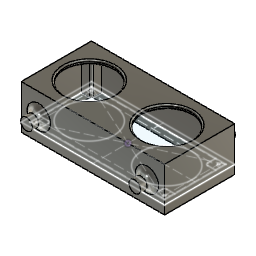
Soporte_EspejoRetrovisor v10 (Autodesk Fusion 360 archive; units mm, degrees)
design "HC-SR04"
Autodesk Fusion 360 part; units mm, degrees
sketch "Boceto1" plane through (0, 0, 0) normal (0, 0, 1) x (1, 0, 0)
  line L0 (22.75, 10.25) -> (-22.75, 10.25)
  line L1 (-22.75, 10.25) -> (-22.75, -10.25)
  line L2 (-22.75, -10.25) -> (22.75, -10.25)
  line L3 (22.75, -10.25) -> (22.75, 10.25)
  line L4 (22.75, 10.25) -> (-22.75, -10.25) construction
  line L5 (-22.75, 10.25) -> (22.75, -10.25) construction
  line L6 (-22.75, -8.5) -> (22.75, -8.5) construction
  line L7 (-21.75, 10.25) -> (-21.75, -10.25) construction
  line L8 (21.75, 10.25) -> (21.75, -10.25) construction
  line L9 (-22.75, 8.5) -> (22.75, 8.5) construction
  circle A0 centre (13.25, 0) radius 8.5
  circle A1 centre (-21.75, 9.25) radius 1 construction
  circle A2 centre (-21.75, 9.25) radius 0.5
  line L10 (12.75, 6.5) -> (22.75, 6.5) construction
  line L11 (0, 10.25) -> (0, -10.25) construction
  circle A3 centre (-13.25, 0) radius 8.5
  line L12 (-22.75, 0) -> (22.75, 0) construction
  line L13 (-22.75, 7.75) -> (22.75, 7.75) construction
  line L14 (-5.0036, 6) -> (5.0036, 6)
  arc A4 (5.0036, 6) -> (5.0036, 9.5) centre (5.0036, 7.75) ccw
  line L15 (5.0036, 9.5) -> (-5.0036, 9.5)
  arc A5 (-5.0036, 9.5) -> (-5.0036, 6) centre (-5.0036, 7.75) ccw
  line L16 (-5.0036, 7.75) -> (5.0036, 7.75) construction
  circle A6 centre (21.75, 9.25) radius 0.5
  circle A7 centre (21.75, 9.25) radius 1 construction
  circle A8 centre (-21.75, -9.25) radius 0.5
  circle A9 centre (-21.75, -9.25) radius 1 construction
  circle A10 centre (21.75, -9.25) radius 1 construction
  circle A11 centre (21.75, -9.25) radius 0.5
  line L17 (-5.0036, -6) -> (5.0036, -6)
  arc A12 (-5.0036, -6) -> (-5.0036, -9.5) centre (-5.0036, -7.75) ccw
  line L18 (5.0036, -9.5) -> (-5.0036, -9.5)
  arc A13 (5.0036, -9.5) -> (5.0036, -6) centre (5.0036, -7.75) ccw
  dimension "d1" = 45.5
  dimension "d2" = 20.5
  dimension "d4" = 1.75
  dimension "d6" = 1
  dimension "d7" = 1
  dimension "d8" = 1.75
  dimension "d9" = 8.5
  dimension "d23" = 1
  dimension "d24" = -0.5
  dimension "d135" = 2.5
  dimension "d136" = 3.5
  constraint horizontal L0
  constraint perpendicular L0 L1
  constraint parallel L0 L2
  constraint parallel L1 L3
  constraint coincident L4 origin
  constraint coincident L5 origin
  constraint coincident L1 L6.start
  constraint coincident L3 L6.end
  constraint perpendicular L3 L6
  constraint coincident L0 L7.start
  constraint coincident L2 L7.end
  constraint perpendicular L2 L7
  constraint coincident L0 L8.start
  constraint coincident L2 L8.end
  constraint perpendicular L2 L8
  constraint coincident L1 L9.start
  constraint coincident L3 L9.end
  constraint perpendicular L3 L9
  constraint tangent L8 A0
  constraint tangent L6 A0
  constraint tangent L0 A1
  constraint tangent L1 A1
  constraint coincident L3 L10.end
  constraint perpendicular L3 L10
  constraint midpoint L0 L11.start
  constraint midpoint L2 L11.end
  constraint symmetric A0 L11 A3
  constraint midpoint L1 L12.start
  constraint midpoint L3 L12.end
  constraint coincident L1 L13.start
  constraint coincident L3 L13.end
  constraint perpendicular L3 L13
  constraint tangent L14 A4
  constraint tangent A4 L15
  constraint parallel L14 L15
  constraint tangent L15 A5
  constraint tangent L14 A5
  constraint perpendicular L11 L16
  constraint coincident L13 A5.centre
  constraint midpoint L13 L16
  constraint symmetric A1 L11 A7
  constraint symmetric A2 L11 A6
  constraint symmetric A1 L12 A9
  constraint symmetric A2 L12 A8
  constraint symmetric L12 A6 A11
  constraint symmetric L12 A7 A10
  constraint symmetric L12 L14.start L17.start
  constraint symmetric L12 L14.end L17.end
  constraint symmetric L12 A4.end L18.start
  constraint symmetric L12 L15.end A12.end
  constraint symmetric L12 A4 A13
  constraint symmetric L12 A5 A12
  measures "d1" distance of L1.end L2.end
  measures "d2" distance of L0.end L1.end
  measures "d4" distance of L2.end L6.end
  measures "d6" distance of L0.end L7.start
  measures "d7" distance of L0.start L8.start
  measures "d8" distance of L0.start L9.end
  measures "d9" radius of A0
  measures "d23" radius of A1
  measures "d135" distance of L0 L13
  measures "d136" diameter of A4
extrude "Extruir5" add sketch "Boceto1" along normal blind 1.6 makes body 1
extrude "Extruir29" add sketch "Boceto1" along normal blind 14 contours A0 | A3 bodies 1
extrude "Extruir30" add sketch "Boceto1" along normal blind 5 contours L14 A4 L15 A5 bodies 1
sketch "Boceto3" plane through (0, 0, 1.6) normal (0, 0, 1) x (-1, 0, 0)
  line L0 (23, -10.5) -> (-23, -10.5)
  line L1 (-23, -10.5) -> (-23, 10.5)
  line L2 (-23, 10.5) -> (23, 10.5)
  line L3 (23, 10.5) -> (23, -10.5)
  line L4 (23, -10.5) -> (-23, 10.5) construction
  line L5 (-23, -10.5) -> (23, 10.5) construction
  line L6 (22.75, -10.25) -> (-22.75, -10.25) construction
  line L7 (-22.75, -10.25) -> (-22.75, 10.25) construction
  line L8 (-22.75, 10.25) -> (22.75, 10.25) construction
  line L9 (22.75, 10.25) -> (22.75, -10.25) construction
  circle A0 centre (21.75, -9.25) radius 1 construction
  circle A1 centre (21.75, -9.25) radius 0.35
  line L10 (-24.5, 12) -> (24.5, 12)
  line L11 (24.5, 12) -> (24.5, -12)
  line L12 (24.5, -12) -> (-24.5, -12)
  line L13 (-24.5, -12) -> (-24.5, 12)
  line L14 (23, -10.5) -> (19.5, -10.5)
  line L15 (19.5, -10.5) -> (19.5, -7.75)
  line L16 (20.25, -7) -> (23, -7)
  line L17 (23, -7) -> (23, -10.5)
  line L18 (22.75, -8.5) -> (-22.75, -8.5) construction
  line L19 (22.75, 8.5) -> (-22.75, 8.5) construction
  line L20 (-21.75, 10.25) -> (-21.75, -10.25) construction
  line L21 (21.75, 10.25) -> (21.75, -10.25) construction
  circle A2 centre (13.25, 0) radius 8.5
  line L22 (24.5, 0) -> (-24.5, 0) construction
  line L23 (0, -12) -> (0, 12) construction
  arc A3 (20.25, -7) -> (19.5, -7.75) centre (20.25, -7.75) ccw
  line L24 (-19.5, -10.5) -> (-19.5, -7.75)
  arc A4 (-19.5, -7.75) -> (-20.25, -7) centre (-20.25, -7.75) ccw
  line L25 (-20.25, -7) -> (-23, -7)
  circle A5 centre (-21.75, -9.25) radius 0.35
  circle A6 centre (-13.25, 0) radius 8.5
  line L26 (19.5, 10.5) -> (19.5, 7.75)
  arc A7 (19.5, 7.75) -> (20.25, 7) centre (20.25, 7.75) ccw
  line L27 (20.25, 7) -> (23, 7)
  circle A8 centre (21.75, 9.25) radius 0.35
  circle A9 centre (-21.75, 9.25) radius 0.35
  line L28 (-19.5, 10.5) -> (-19.5, 7.75)
  arc A10 (-20.25, 7) -> (-19.5, 7.75) centre (-20.25, 7.75) ccw
  line L29 (-20.25, 7) -> (-23, 7)
  point P0 (19.5, -7)
  dimension "d79" = 46
  dimension "d80" = 21
  dimension "d81" = 0.25
  dimension "d82" = 1
  dimension "d83" = -0.65
  dimension "d87" = -1.5
  dimension "d88" = 3.5
  dimension "d89" = 3.5
  dimension "d90" = 1.75
  dimension "d91" = 1.75
  dimension "d92" = 1
  dimension "d93" = 1
  dimension "d94" = 8.5
  dimension "d95" = 0.75
  constraint horizontal L0
  constraint perpendicular L0 L1
  constraint parallel L0 L2
  constraint parallel L1 L3
  constraint coincident L4 origin
  constraint coincident L5 origin
  constraint tangent L6 A0
  constraint tangent L9 A0
  constraint horizontal L14
  constraint vertical L15
  constraint horizontal L16
  constraint vertical L17
  constraint coincident L9 L18.start
  constraint coincident L7 L18.end
  constraint perpendicular L7 L18
  constraint coincident L9 L19.start
  constraint coincident L7 L19.end
  constraint perpendicular L7 L19
  constraint coincident L8 L20.start
  constraint coincident L6 L20.end
  constraint perpendicular L6 L20
  constraint coincident L8 L21.start
  constraint coincident L6 L21.end
  constraint perpendicular L6 L21
  constraint tangent L21 A2
  constraint tangent L19 A2
  constraint midpoint L11 L22.start
  constraint midpoint L13 L22.end
  constraint midpoint L12 L23.start
  constraint midpoint L10 L23.end
  constraint coincident P0 L15
  constraint coincident P0 L16
  constraint tangent L15 A3
  constraint tangent L16 A3
  constraint symmetric A1 L23 A5
  constraint symmetric L14.end L23 L24.start
  constraint symmetric L16.end L23 L25.end
  constraint symmetric A2 L23 A6
  constraint symmetric L23 L15.end L24.end
  constraint symmetric L23 L16.start A4.end
  constraint symmetric L23 A3 A4
  constraint symmetric A1 L22 A8
  constraint symmetric L14.end L22 L26.start
  constraint symmetric L16.end L22 L27.end
  constraint symmetric L22 L15.end L26.end
  constraint symmetric L22 L16.start A7.end
  constraint symmetric L22 A3 A7
  constraint symmetric L22 L24.start L28.start
  constraint symmetric L22 L24.end L28.end
  constraint symmetric L22 A4.end A10.start
  constraint symmetric L22 A4 A10
  constraint symmetric L22 L25.end L29.end
  constraint symmetric L22 A5 A9
  measures "d79" distance of L0.start L0.end
  measures "d80" distance of L0.end L1.end
  measures "d82" radius of A0
  measures "d88" distance of L14.end P0
  measures "d89" distance of P0 L16.end
  measures "d90" distance of L6 L18
  measures "d91" distance of L8 L19
  measures "d92" distance of L7 L20
  measures "d93" distance of L9 L21
  measures "d94" radius of A2
  measures "d95" radius of A3
extrude "Extruir20" add sketch "Boceto3" along normal blind 12 and the other way blind 3 separate body contours L10 L11 L12 L13 makes body 2
extrude "Extruir21" add sketch "Boceto3" along normal blind 12 contours L0 L3 L14 L15 L16 L17 A3 | L0 L1 L24 A4 L25 | L2 L3 L26 A7 L27 | L1 L2 L28 A10 L29 | A1 | A5 | A8 | A9 bodies 2
extrude "Extruir22" add sketch "Boceto3" along normal blind 1.5 from surface at 10.5 contours L0 L1 L2 L3 L15 L16 A3 L24 A4 L25 L26 A7 L27 L28 A10 L29 bodies 2
extrude "Extruir23" cut sketch "Boceto3" along normal blind 4 contours A1 | A5 | A8 | A9 bodies 2
sketch "Boceto4" plane through (0, -12, 0) normal (0, -1, 0) x (1, 0, 0)
  line L0 (24.5, -1.4) -> (24.5, 13.6)
  line L1 (24.5, 13.6) -> (-24.5, 13.6)
  line L2 (-24.5, 13.6) -> (-24.5, -1.4)
  line L3 (-24.5, -1.4) -> (24.5, -1.4)
  line L4 (-24.5, 6.1) -> (24.5, 6.1) construction
  line L5 (-24.5, 13.6) -> (24.5, 13.6) construction
  line L6 (24.5, 13.6) -> (24.5, -1.4) construction
  line L7 (24.5, -1.4) -> (-24.5, -1.4) construction
  line L8 (-24.5, -1.4) -> (-24.5, 13.6) construction
  line L9 (-20.5, 13.6) -> (-20.5, -1.4) construction
  line L10 (0, 13.6) -> (0, -1.4) construction
  line L11 (-24.5, 8.1) -> (24.5, 8.1) construction
  circle A0 centre (-18.5, 6.1) radius 2
  circle A1 centre (18.5, 6.1) radius 2
  dimension "d151" = 4
  dimension "d154" = 2
  dimension "d155" = 2
  constraint midpoint L2 L4.start
  constraint midpoint L0 L4.end
  constraint horizontal L5
  constraint vertical L6
  constraint horizontal L7
  constraint vertical L8
  constraint coincident L0.start L3.end
  constraint coincident L1.end L2.start
  constraint coincident L5 L9.start
  constraint coincident L7 L9.end
  constraint perpendicular L7 L9
  constraint midpoint L5 L10.start
  constraint midpoint L7 L10.end
  constraint coincident L8 L11.start
  constraint coincident L6 L11.end
  constraint perpendicular L6 L11
  constraint tangent L11 A0
  constraint tangent L9 A0
  constraint symmetric L10 A0 A1
  measures "d151" distance of L8 L9
  measures "d154" distance of L4 L11
  measures "d155" radius of A0
sketch "Boceto5" plane through (0, 12, 0) normal (0, 1, 0) x (-1, 0, 0)
  line L0 (24.5, -1.4) -> (24.5, 13.6)
  line L1 (24.5, 13.6) -> (-24.5, 13.6)
  line L2 (-24.5, 13.6) -> (-24.5, -1.4)
  line L3 (-24.5, -1.4) -> (24.5, -1.4)
  line L4 (-24.5, 13.6) -> (24.5, 13.6) construction
  line L5 (24.5, 13.6) -> (24.5, -1.4) construction
  line L6 (24.5, -1.4) -> (-24.5, -1.4) construction
  line L7 (-24.5, -1.4) -> (-24.5, 13.6) construction
  line L8 (0, 13.6) -> (0, -1.4) construction
  line L9 (-24.5, 6.1) -> (24.5, 6.1) construction
  line L10 (20.5, 13.6) -> (20.5, -1.4) construction
  line L11 (24.5, 8.1) -> (-24.5, 8.1) construction
  circle A0 centre (18.5, 6.1) radius 2
  circle A1 centre (-18.5, 6.1) radius 2
  dimension "d156" = 4
  dimension "d157" = 2
  dimension "d158" = 2
  constraint horizontal L4
  constraint vertical L5
  constraint horizontal L6
  constraint vertical L7
  constraint coincident L0.start L3.end
  constraint coincident L1.end L2.start
  constraint midpoint L1 L8.start
  constraint midpoint L3 L8.end
  constraint midpoint L2 L9.start
  constraint midpoint L5 L9.end
  constraint coincident L1 L10.start
  constraint coincident L6 L10.end
  constraint perpendicular L6 L10
  constraint coincident L5 L11.start
  constraint coincident L2 L11.end
  constraint perpendicular L2 L11
  constraint tangent L11 A0
  constraint tangent L10 A0
  constraint symmetric L8 A0 A1
  measures "d156" distance of L5 L10
  measures "d157" distance of L9 L11
  measures "d158" radius of A0
extrude "Extruir31" add sketch "Boceto5" along normal blind 4.2 contours A0 | A1 bodies 2
extrude "Extruir32" add sketch "Boceto4" along normal blind 4.2 contours A0 | A1 bodies 2
fillet "Empalme3" radius 2 4 edges at (-20.3647, -12, 6.8232) (16.6353, -12, 6.8232) (20.3647, 12, 6.8232) (-16.6353, 12, 6.8232) on bodies 2
fillet "Empalme3" radius 0.5 4 edges at (-5.3252, -3.0737, 13.6) (21.1748, -3.0737, 13.6) (-5.3252, -3.0737, 12.1) (21.1748, -3.0737, 12.1) on bodies 2
hidden bodies 1
named bodies: "HC-SR04", "Carcasa_HC-SR04"
